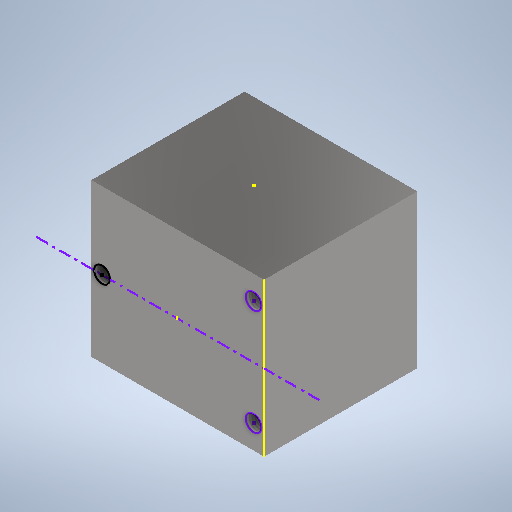
# Autodesk Inventor part: Camera
Saved by Autodesk Inventor 2025.1 (Build 291241000, 241)
## iProperties
Created: 2024-09-22
Part Number: Camera
Material: Steel, Alloy
Document SubType Name: Modeling
Designer: JuhenFW
Density: 7.73 g/cm^3
Appearance: Semi-Polished
Author: JuhenFW
Autodesk Inventor part; units mm, degrees
ref_plane "YZ Plane" through (0, 0, 0) normal (1, 0, 0) x (0, 1, 0)
ref_plane "XZ Plane" through (0, 0, 0) normal (0, 1, 0) x (-1, 0, 0)
sketch "Sketch1" plane through (0, 0, 0) normal (0, 0, 1) x (1, 0, 0)
  line L0 (-16.35, -14.5) -> (16.35, -14.5)
  line L1 (16.35, -14.5) -> (16.35, 14.5)
  line L2 (16.35, 14.5) -> (-16.35, 14.5)
  line L3 (-16.35, 14.5) -> (-16.35, -14.5)
  line L4 (-16.35, -14.5) -> (16.35, 14.5) construction
  line L5 (16.35, -14.5) -> (-16.35, 14.5) construction
  point P0 (0, 0)
  dimension "d0" = 32.7
  dimension "d1" = 29
  constraints: 12 end point, 2 midpoint, 2 parallel, 1 horizontal, 1 perpendicular
  measures "d0" distance of L2.end L1.end
  measures "d1" distance between parallel lines of L0 L2
extrude "Extrusion1" add sketch "Sketch1" along normal mid plane 29
sketch "Sketch2" plane through (0, 0, 14.5) normal (0, 0, 1) x (1, 0, 0)
  circle A0 centre (14.35, 10) radius 1.5
  circle A1 centre (14.35, -10) radius 1.5
  circle A2 centre (-14.35, 0) radius 1.5
  line L0 (16.35, -14.5) -> (16.35, 14.5) projected
  line L1 (-26.8046, 0) -> (27.4172, 0)
  point P0 (0, 0)
  dimension "d4" = 3
  dimension "d5" = 3
  dimension "d6" = 3
  dimension "d7" = 20
  dimension "d8" = 2
  dimension "d9" = 28.7
  constraints: 3 centre point, 2 end point, 1 horizontal, 1 horizontal alignment, 1 symmetric about line, 1 vertical alignment
  measures "d4" diameter of A0
  measures "d5" diameter of A1
  measures "d6" diameter of A2
  measures "d7" distance of A1.centre A0.centre
  measures "d8" distance from line of L0 A0.centre
  measures "d9" horizontal distance of A2.centre A0.centre
extrude "Extrusion2" cut sketch "Sketch2" against normal blind 4
thread "Thread1" size "M3x0.5" class "6H" standard "ANSI Metric M Profile" length 5
thread "Thread2" size "M3x0.5" class "6H" standard "ANSI Metric M Profile" length 5
thread "Thread3" size "M3x0.5" class "6H" standard "ANSI Metric M Profile" length 5
sketch "Sketch3" plane through (0, 0, -14.5) normal (0, 0, -1) x (-1, 0, 0)
  point P0 (0, 0)
sketch "Sketch4" plane through (-16.35, 14.5, 14.5) normal (0, 1, 0) x (1, 0, 0)
  point P0 (16.35, 14.5)
ref_plane "Work Plane2" through (0, 0, -14.5) normal (0, 0, 1) x (1, 0, 0)
sketch "Sketch6" plane through (0, 0, -14.5) normal (0, 0, 1) x (1, 0, 0)
  circle A0 centre (-14.3431, 0) radius 1.5
  circle A1 centre (14.35, -10) radius 1.5 projected
  circle A2 centre (14.35, -10) radius 1.5
  circle A3 centre (14.35, 9.9933) radius 1.5
  point P0 (0, 0)
  dimension "d20" = 3
  dimension "d21" = 3
  dimension "d22" = 3
  constraints: 3 centre point, 1 coincident
  measures "d20" diameter of A0
  measures "d21" diameter of A2
  measures "d22" diameter of A3
sketch "Sketch7" plane through (0, 0, -14.5) normal (0, 0, -1) x (-1, 0, 0)
  point P0 (0, 0)
extrude "Extrusion3" cut sketch "Sketch6" along normal blind 3
thread "Thread4" size "M3x0.5" class "6H" standard "ANSI Metric M Profile" length 5
thread "Thread5" size "M3x0.5" class "6H" standard "ANSI Metric M Profile" length 5
thread "Thread6" size "M3x0.5" class "6H" standard "ANSI Metric M Profile" length 5
equation "\"d23\" = d20"
body "Solid1"
